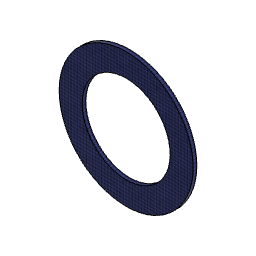
Extension Piece v2 (Autodesk Fusion 360 archive; units mm, degrees)
design "average flange blue seal"
Autodesk Fusion 360 part; units mm, degrees
cylinder "CylinderPrimitive1" add diameter 76 height 1.5875 placed x (1, 0, 0) y (0, 0, -1) z (0, 1, 0) at (0, 0, 0)
hole "Hole1" at (0, 0, 0) direction (0, 1, 0) diameter 48 depth 20 tip angle 180
extrude "Extrude1" add 1 faces at (33.1695, 1.5875, 2.4857) along direction (0, 1, 0) blind 0.4125
extrude "Extrude2" cut 1 faces at (33.1695, 0, 2.4857) along direction (0, 1, 0) blind 0.876
extrude "Extrude3" add 1 faces at (33.1695, 0.876, 2.4857) along direction (0, -1, 0) blind 0.876
sketch "Sketch2" plane through (0, 0, 0) normal (0, -1, 0) x (1, 0, 0)
  circle A0 centre (0, 0) radius 24
  circle A1 centre (0, 0) radius 38
  circle A2 centre (0, 0) radius 36.5
  dimension "d13" = 73
  constraint coincident A0.centre A1.centre
  measures "d13" diameter of A2
extrude "Extrude4" cut sketch "Sketch2" against normal blind 2 contours A1
